to modle anicies-dup (Autodesk Fusion 360 design; units mm, degrees)
Autodesk Fusion 360 part; units mm, degrees
sketch "Sketch1" plane through (0, 0, 0) normal (0, 0, 1) x (1, 0, 0)
  line L0 (-22.9576, -22.2881) -> (29.9321, -22.2881)
  arc A0 (29.9321, -22.2881) -> (29.9321, -10.0567) centre (29.9321, -16.1724) ccw
  line L1 (29.9321, -10.0567) -> (-22.9576, -10.0567)
  arc A1 (-22.9576, 2.1746) -> (-22.9576, -10.0567) centre (-22.9576, -3.941) ccw
  line L2 (-22.9576, 2.1746) -> (29.9321, 2.1746)
  line L3 (3.4873, -22.2881) -> (3.4873, 2.1746) construction
  constraint horizontal L0
  constraint tangent L0 A0
  constraint tangent A0 L1
  constraint parallel L0 L1
  constraint tangent L1 A1
  constraint tangent A1 L2
  constraint horizontal L2
  constraint coincident L0 L3.start
  constraint coincident L2 L3.end
  constraint perpendicular L2 L3
  constraint midpoint L1 L3
  constraint equal L0 L2
  constraint equal L1 L2
surface "Extrude1" add extruded along (0, 0, 1) between 0 and 10 path "Sketch1" along L0 A0 L1 A1 L2 makes body 1
thicken "Thicken1" add thickness 0.1 25 faces at (-5.3277, 2.1746, 3.3333) (-24.4667, -9.8676, 6.6667) (12.3022, -10.0567, 3.3333) (30.5411, -10.0871, 3.3333) (-5.3277, -22.2881, 3.3333) (-24.4667, -9.8676, 6.6667) (12.3022, -10.0567, 3.3333) (30.5411, -10.0871, 3.3333) (-5.3277, -22.2881, 3.3333) (-5.3277, 2.1746, 3.3333) (12.3022, -10.0567, 3.3333) (30.5411, -10.0871, 3.3333) (-5.3277, -22.2881, 3.3333) (-24.4667, -9.8676, 6.6667) (-5.3277, 2.1746, 3.3333) (30.5411, -10.0871, 3.3333) (-5.3277, -22.2881, 3.3333) (12.3022, -10.0567, 3.3333) (-24.4667, -9.8676, 6.6667) (-5.3277, 2.1746, 3.3333) (-5.3277, -22.2881, 3.3333) (30.5411, -10.0871, 3.3333) (12.3022, -10.0567, 3.3333) (-24.4667, -9.8676, 6.6667) (-5.3277, 2.1746, 3.3333) separate body on bodies 1 makes body 2
hidden bodies 1
